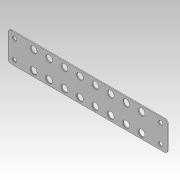
# Autodesk Inventor part: SolenoidBracket
Saved by Autodesk Inventor 2020 (Build 240168000, 168)
## iProperties
Created: 2021-08-03
Part Number: SolenoidBracket
Material: Generic
Document SubType Name: Modeling
Designer: DDeGo
Density: 1 g/cm^3
Appearance: Default
Author: DDeGo
Autodesk Inventor part; units mm, degrees
ref_plane "YZ Plane" through (0, 0, 0) normal (1, 0, 0) x (0, 1, 0)
ref_plane "XZ Plane" through (0, 0, 0) normal (0, 1, 0) x (-1, 0, 0)
sketch "Sketch1" plane through (0, 0, 0) normal (0, 0, 1) x (1, 0, 0)
  line L0 (0, 0) -> (0, 12.5) construction
  line L1 (-10.5, 4.25) -> (10.5, 4.25) construction
  line L2 (10.5, 4.25) -> (10.5, 20.75) construction
  line L3 (10.5, 20.75) -> (-10.5, 20.75) construction
  line L4 (-10.5, 20.75) -> (-10.5, 4.25) construction
  line L5 (-10.5, 4.25) -> (10.5, 20.75) construction
  line L6 (10.5, 4.25) -> (-10.5, 20.75) construction
  circle A0 centre (0, 12.5) radius 4.5
  line L7 (0, 0) -> (-23.3599, 0) construction
  line L8 (0, 0) -> (0, -12.5) construction
  line L9 (-10.5, -4.25) -> (10.5, -4.25) construction
  line L10 (10.5, -4.25) -> (10.5, -20.75) construction
  line L11 (10.5, -20.75) -> (-10.5, -20.75) construction
  line L12 (-10.5, -20.75) -> (-10.5, -4.25) construction
  line L13 (-10.5, -4.25) -> (10.5, -20.75) construction
  line L14 (10.5, -4.25) -> (-10.5, -20.75) construction
  circle A1 centre (0, -12.5) radius 4.5
  line L15 (10.5, 4.25) -> (31.5, 4.25) construction
  line L16 (21, 0) -> (21, 12.5) construction
  circle A2 centre (21, 12.5) radius 4.5
  line L17 (31.5, 4.25) -> (31.5, 20.75) construction
  line L18 (31.5, 4.25) -> (10.5, 20.75) construction
  line L19 (31.5, 20.75) -> (10.5, 20.75) construction
  line L20 (10.5, 20.75) -> (10.5, 4.25) construction
  line L21 (10.5, 4.25) -> (31.5, 20.75) construction
  line L22 (10.5, -4.25) -> (31.5, -4.25) construction
  line L23 (21, 0) -> (21, -12.5) construction
  circle A3 centre (21, -12.5) radius 4.5
  line L24 (31.5, -20.75) -> (10.5, -20.75) construction
  line L25 (10.5, -20.75) -> (10.5, -4.25) construction
  line L26 (10.5, -4.25) -> (31.5, -20.75) construction
  line L27 (31.5, -4.25) -> (31.5, -20.75) construction
  line L28 (31.5, -4.25) -> (10.5, -20.75) construction
  line L29 (31.5, 4.25) -> (52.5, 4.25) construction
  line L30 (42, 0) -> (42, 12.5) construction
  circle A4 centre (42, 12.5) radius 4.5
  line L31 (52.5, 4.25) -> (52.5, 20.75) construction
  line L32 (52.5, 4.25) -> (31.5, 20.75) construction
  line L33 (52.5, 20.75) -> (31.5, 20.75) construction
  line L34 (31.5, 20.75) -> (31.5, 4.25) construction
  line L35 (31.5, 4.25) -> (52.5, 20.75) construction
  line L36 (31.5, -4.25) -> (52.5, -4.25) construction
  line L37 (42, 0) -> (42, -12.5) construction
  circle A5 centre (42, -12.5) radius 4.5
  line L38 (52.5, -20.75) -> (31.5, -20.75) construction
  line L39 (31.5, -20.75) -> (31.5, -4.25) construction
  line L40 (31.5, -4.25) -> (52.5, -20.75) construction
  line L41 (52.5, -4.25) -> (52.5, -20.75) construction
  line L42 (52.5, -4.25) -> (31.5, -20.75) construction
  line L43 (52.5, 4.25) -> (73.5, 4.25) construction
  line L44 (63, 0) -> (63, 12.5) construction
  circle A6 centre (63, 12.5) radius 4.5
  line L45 (73.5, 4.25) -> (73.5, 20.75) construction
  line L46 (73.5, 4.25) -> (52.5, 20.75) construction
  line L47 (73.5, 20.75) -> (52.5, 20.75) construction
  line L48 (52.5, 20.75) -> (52.5, 4.25) construction
  line L49 (52.5, 4.25) -> (73.5, 20.75) construction
  line L50 (52.5, -4.25) -> (73.5, -4.25) construction
  line L51 (63, 0) -> (63, -12.5) construction
  circle A7 centre (63, -12.5) radius 4.5
  line L52 (73.5, -20.75) -> (52.5, -20.75) construction
  line L53 (52.5, -20.75) -> (52.5, -4.25) construction
  line L54 (52.5, -4.25) -> (73.5, -20.75) construction
  line L55 (73.5, -4.25) -> (73.5, -20.75) construction
  line L56 (73.5, -4.25) -> (52.5, -20.75) construction
  line L57 (73.5, 4.25) -> (94.5, 4.25) construction
  line L58 (84, 0) -> (84, 12.5) construction
  circle A8 centre (84, 12.5) radius 4.5
  line L59 (94.5, 4.25) -> (94.5, 20.75) construction
  line L60 (94.5, 4.25) -> (73.5, 20.75) construction
  line L61 (94.5, 20.75) -> (73.5, 20.75) construction
  line L62 (73.5, 20.75) -> (73.5, 4.25) construction
  line L63 (73.5, 4.25) -> (94.5, 20.75) construction
  line L64 (73.5, -4.25) -> (94.5, -4.25) construction
  line L65 (84, 0) -> (84, -12.5) construction
  circle A9 centre (84, -12.5) radius 4.5
  line L66 (94.5, -20.75) -> (73.5, -20.75) construction
  line L67 (73.5, -20.75) -> (73.5, -4.25) construction
  line L68 (73.5, -4.25) -> (94.5, -20.75) construction
  line L69 (94.5, -4.25) -> (94.5, -20.75) construction
  line L70 (94.5, -4.25) -> (73.5, -20.75) construction
  line L71 (94.5, 4.25) -> (115.5, 4.25) construction
  line L72 (105, 0) -> (105, 12.5) construction
  circle A10 centre (105, 12.5) radius 4.5
  line L73 (115.5, 4.25) -> (115.5, 20.75) construction
  line L74 (115.5, 4.25) -> (94.5, 20.75) construction
  line L75 (115.5, 20.75) -> (94.5, 20.75) construction
  line L76 (94.5, 20.75) -> (94.5, 4.25) construction
  line L77 (94.5, 4.25) -> (115.5, 20.75) construction
  line L78 (94.5, -4.25) -> (115.5, -4.25) construction
  line L79 (105, 0) -> (105, -12.5) construction
  circle A11 centre (105, -12.5) radius 4.5
  line L80 (115.5, -20.75) -> (94.5, -20.75) construction
  line L81 (94.5, -20.75) -> (94.5, -4.25) construction
  line L82 (94.5, -4.25) -> (115.5, -20.75) construction
  line L83 (115.5, -4.25) -> (115.5, -20.75) construction
  line L84 (115.5, -4.25) -> (94.5, -20.75) construction
  line L85 (115.5, 4.25) -> (136.5, 4.25) construction
  line L86 (126, 0) -> (126, 12.5) construction
  circle A12 centre (126, 12.5) radius 4.5
  line L87 (136.5, 4.25) -> (136.5, 20.75) construction
  line L88 (136.5, 4.25) -> (115.5, 20.75) construction
  line L89 (136.5, 20.75) -> (115.5, 20.75) construction
  line L90 (115.5, 20.75) -> (115.5, 4.25) construction
  line L91 (115.5, 4.25) -> (136.5, 20.75) construction
  line L92 (115.5, -4.25) -> (136.5, -4.25) construction
  line L93 (126, 0) -> (126, -12.5) construction
  circle A13 centre (126, -12.5) radius 4.5
  line L94 (136.5, -20.75) -> (115.5, -20.75) construction
  line L95 (115.5, -20.75) -> (115.5, -4.25) construction
  line L96 (115.5, -4.25) -> (136.5, -20.75) construction
  line L97 (136.5, -4.25) -> (136.5, -20.75) construction
  line L98 (136.5, -4.25) -> (115.5, -20.75) construction
  line L99 (136.5, 4.25) -> (157.5, 4.25) construction
  line L100 (147, 0) -> (147, 12.5) construction
  circle A14 centre (147, 12.5) radius 4.5
  line L101 (157.5, 4.25) -> (157.5, 20.75) construction
  line L102 (157.5, 4.25) -> (136.5, 20.75) construction
  line L103 (157.5, 20.75) -> (136.5, 20.75) construction
  line L104 (136.5, 20.75) -> (136.5, 4.25) construction
  line L105 (136.5, 4.25) -> (157.5, 20.75) construction
  line L106 (136.5, -4.25) -> (157.5, -4.25) construction
  line L107 (147, 0) -> (147, -12.5) construction
  circle A15 centre (147, -12.5) radius 4.5
  line L108 (157.5, -20.75) -> (136.5, -20.75) construction
  line L109 (136.5, -20.75) -> (136.5, -4.25) construction
  line L110 (136.5, -4.25) -> (157.5, -20.75) construction
  line L111 (157.5, -4.25) -> (157.5, -20.75) construction
  line L112 (157.5, -4.25) -> (136.5, -20.75) construction
  line L113 (-35, 19.75) -> (182, 19.75)
  line L114 (182, 19.75) -> (182, -19.75)
  line L115 (182, -19.75) -> (-35, -19.75)
  line L116 (-35, -19.75) -> (-35, 19.75)
  line L117 (-35, 0) -> (-26, 0) construction
  line L118 (-26, 0) -> (-26, 12.5) construction
  line L119 (-26, 0) -> (-26, -12.5) construction
  line L120 (182, 0) -> (173, 0) construction
  line L121 (173, 0) -> (173, 12.5) construction
  line L122 (173, 0) -> (173, -12.5) construction
  circle A16 centre (-26, 12.5) radius 2.75
  circle A17 centre (-26, -12.5) radius 2.75
  circle A18 centre (173, 12.5) radius 2.75
  circle A19 centre (173, -12.5) radius 2.75
  dimension "d0" = 12.5
  dimension "d1" = 21
  dimension "d2" = 16.5
  dimension "d3" = 9
  dimension "d6" = 21
  dimension "d11" = 1
  dimension "d12" = 1
  dimension "d17" = 26
  dimension "d18" = 25
  dimension "d19" = 5.5
  dimension "d20" = 217
  dimension "d29" = 9
  dimension "d30" = 26
  constraints: 246 end point, 34 midpoint, 20 centre point, 20 coincident, 6 horizontal, 6 symmetric about line, 4 equal length, 4 parallel, 4 perpendicular, 3 equal radius, 3 vertical, 204 other
  measures "d0" distance of L0.start L0.end
  measures "d1" distance of L2.end L3.end
  measures "d2" distance of L1.end L2.end
  measures "d3" diameter of A0
  measures "d6" distance of L0.start L16.start
  measures "d11" distance between parallel lines of L3 L113
  measures "d12" distance between parallel lines of L11 L115
  measures "d17" distance from line of L0.end L118
  measures "d18" distance of L119.end L118.end
  measures "d19" diameter of A16
  measures "d20" distance between parallel lines of L114 L116
  measures "d29" distance between parallel lines of L116 L118
  measures "d30" distance between parallel lines of L121 L100
extrude "Extrusion1" add sketch "Sketch1" along normal blind 1.2
ref_plane "Work Plane1" through (0, 0, 0) normal (0, 1, 0) x (-1, 0, 0)
sketch "Sketch2" plane through (0, 0, 0) normal (0, 1, 0) x (-1, 0, 0)
  line L0 (35, 0) -> (-182, 0) construction
  line L1 (35, 0) -> (32, 0) construction
  line L2 (32, 0) -> (3.6436, -5)
  line L3 (3.6436, -5) -> (-150.6436, -5)
  line L4 (-150.6436, -5) -> (-179, 0)
  line L5 (-179, 0) -> (-182, 0) construction
  line L6 (-179, 0) -> (32, 0)
  point P0 (0, 0)
  dimension "d21" = 3
  dimension "d22" = 5
  dimension "d31" = 10
  constraints: 12 end point, 2 equal length, 1 collinear, 1 horizontal, 1 parallel, 1 point on line
  measures "d21" distance of L0.start L1.end
  measures "d22" distance between parallel lines of L0 L3
  measures "d31" angle of L0 L2
extrude "Extrusion2" add sketch "Sketch2" along normal mid plane 3
fillet "Fillet1" radius 2 2 edges at (73.5, 1.5, 0) (73.5, -1.5, 0)
fillet "Fillet1" radius 20 2 edges at (-3.6436, 0, -5) (150.6436, 0, -5)
fillet "Fillet2" radius 0.5 14 edges at (-3.6369, 1.5, -4.9239) (-13.0121, 1.5, -3.3481) (-28.6778, 2.0858, -0.5858) (150.6369, 1.5, -4.9239) (160.0121, 1.5, -3.3481) (175.6778, 2.0858, -0.5858) (73.5, 1.5, -5) (150.6369, -1.5, -4.9239) (160.0121, -1.5, -3.3481) (175.6778, -2.0858, -0.5858) (-3.6369, -1.5, -4.9239) (-13.0121, -1.5, -3.3481) (-28.6778, -2.0858, -0.5858) (73.5, -1.5, -5)
fillet "Fillet3" radius 4 4 edges at (-35, -19.75, 0.6) (-35, 19.75, 0.6) (182, -19.75, 0.6) (182, 19.75, 0.6)
equation "\"d6\" = d1"
equation "\"d30\" = d17"
body "Solid1"
